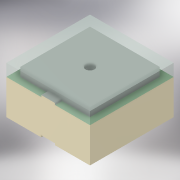
# Autodesk Inventor part: 13360-30xxVE
Saved by Autodesk Inventor 2019 (Build 230136000, 136)
## iProperties
Created: 2016-06-07
Part Number: 13360-30xxVE
Material: ABS Plastic
Document SubType Name: Modeling
Designer: sawaiz
Density: 1.06 g/cm^3
Appearance: Smooth - White
Author: sawaiz
Autodesk Inventor part; units mm, degrees
ref_plane "YZ Plane" through (0, 0, 0) normal (1, 0, 0) x (0, 1, 0)
ref_plane "XZ Plane" through (0, 0, 0) normal (0, 1, 0) x (-1, 0, 0)
ref_plane "XY Plane" through (0, 0, 0) normal (0, 0, 1) x (1, 0, 0)
sketch "Sketch1" plane through (0, 0, 0) normal (0, 1, 0) x (-1, 0, 0)
  line L0 (1.2, 1.2) -> (-1.2, 1.2)
  line L1 (-1.2, 1.2) -> (-1.2, -1.2)
  line L2 (-1.2, -1.2) -> (1.2, -1.2)
  line L3 (1.2, -1.2) -> (1.2, 1.2)
  line L4 (1.2, 1.2) -> (-1.2, -1.2) construction
  line L5 (-1.2, 1.2) -> (1.2, -1.2) construction
  point P0 (0, 0)
  dimension "d0" = 2.4
  dimension "d1" = 2.4
  constraints: 12 end point, 2 midpoint, 2 parallel, 1 horizontal, 1 perpendicular
  measures "d0" distance of L2.end L1.end
  measures "d1" distance of L1.end L0.end
extrude "Extrusion1" add sketch "Sketch1" along normal blind 1
sketch "Sketch2" plane through (0, 1, 0) normal (0, 1, 0) x (1, 0, 0)
  line L0 (1, -1) -> (-1, -1)
  line L1 (-1, -1) -> (-1, 1)
  line L2 (-1, 1) -> (1, 1)
  line L3 (1, 1) -> (1, -1)
  line L4 (1, -1) -> (-1, 1) construction
  line L5 (-1, -1) -> (1, 1) construction
  point P0 (0, 0)
  dimension "d4" = 2
  dimension "d5" = 2
  constraints: 12 end point, 2 midpoint, 2 parallel, 1 horizontal, 1 perpendicular
  measures "d4" distance of L1.end L2.end
  measures "d5" distance of L0.end L1.end
extrude "Extrusion2" add sketch "Sketch2" along normal blind 0.25 separate body
sketch "Sketch8" plane through (0, 1, 0) normal (0, 1, 0) x (1, 0, 0)
  line L0 (-1.2, -1.2) -> (1.2, -1.2) projected
  line L1 (1.2, -1.2) -> (1.2, 1.2) projected
  line L2 (1.2, 1.2) -> (-1.2, 1.2) projected
  line L3 (-1.2, 1.2) -> (-1.2, -1.2) projected
  line L4 (-1, -1) -> (1, -1) projected
  line L5 (-0.2, -1.2) -> (0.2, -1.2)
  line L6 (0.2, -1.2) -> (0.2, -1)
  line L7 (0.2, -1) -> (-0.2, -1)
  line L8 (-0.2, -1) -> (-0.2, -1.2)
  point P0 (0, 0)
  point P1 (0, -1)
  point P2 (0, -1.2)
  dimension "d49" = 0.4
  constraints: 8 end point, 3 midpoint, 2 parallel, 2 point on line, 1 horizontal, 1 perpendicular
  measures "d49" distance between parallel lines of L8 L6
extrude "Extrusion6" add sketch "Sketch8" along normal blind 0.05 contours L8 L4 L6 L0 bodies 1
sketch "Sketch3" plane through (0, 1, 0) normal (0, 1, 0) x (1, 0, 0)
  line L0 (-1.2, -1.2) -> (-0.2, -1.2) projected
  line L1 (1.2, -1.2) -> (1.2, 1.2) projected
  line L2 (1.2, 1.2) -> (-1.2, 1.2) projected
  line L3 (-1.2, 1.2) -> (-1.2, -1.2) projected
  line L4 (-1, -1) -> (1, -1) projected
  line L5 (1, -1) -> (1, 1) projected
  line L6 (1, 1) -> (-1, 1) projected
  line L7 (-1, 1) -> (-1, -1) projected
  line L8 (0.2, -1) -> (0.2, -1.2) projected
  line L9 (0.2, -1.2) -> (1.2, -1.2) projected
  line L10 (-0.2, -1.2) -> (-0.2, -1) projected
  line L11 (-0.2, -1) -> (0.2, -1) projected
  point P0 (0, 0)
extrude "Extrusion3" add sketch "Sketch3" along normal blind 0.35 separate body contours L3 L2 L1 L9 L8 L4 L5 L6 L7 L10 L0
sketch "Sketch9" plane through (0, 1.05, 0) normal (0, 1, 0) x (1, 0, 0)
  point P0 (0, 0)
sketch "Sketch10" plane through (0, 1.35, 0) normal (0, 1, 0) x (1, 0, 0)
  line L0 (-0.2, -1.2) -> (0.2, -1.2) projected
  line L1 (0.2, -1.2) -> (0.2, -1) projected
  line L2 (0.2, -1) -> (-0.2, -1) projected
  line L3 (-0.2, -1) -> (-0.2, -1.2) projected
  point P0 (0, 0)
extrude "Extrusion7" add sketch "Sketch10" against normal up to surface (0.3 mm away) bodies 3
sketch "Sketch5" plane through (0, 1.25, 0) normal (0, 1, 0) x (1, 0, 0)
  point P0 (0, 0)
  point P1 (0, 0)
  constraints: 1 coincident
hole "Hole1" at (0, 1.25, 0) direction (0, -1, 0) diameter 0.254 depth 0.1 tip angle 118 bodies 2
sketch "Sketch4" plane through (0, 1.35, 0) normal (0, 1, 0) x (1, 0, 0)
  line L0 (-1, -1) -> (-1, 1) projected
  line L1 (-1, 1) -> (1, 1) projected
  line L2 (1, 1) -> (1, -1) projected
  line L3 (1, -1) -> (-1, -1) projected
  line L4 (1.2, -1.2) -> (1.2, 1.2) projected
  line L5 (1.2, 1.2) -> (-1.2, 1.2) projected
  line L6 (-1.2, 1.2) -> (-1.2, -1.2) projected
  line L7 (-1.2, -1.2) -> (1.2, -1.2) projected
  point P0 (0, 0)
extrude "Extrusion4" add sketch "Sketch4" against normal up to surface (0.1 mm away) contours L0 L1 L2 L3 bodies 3
sketch "Sketch6" plane through (0, 0, 0) normal (0, -1, 0) x (1, 0, 0)
  line L0 (0.6, 0.6) -> (-0.6, 0.6)
  line L1 (-0.6, 0.6) -> (-0.6, -0.6)
  line L2 (-0.6, -0.6) -> (0.6, -0.6)
  line L3 (0.6, -0.6) -> (0.6, 0.6)
  line L4 (0.6, 0.6) -> (-0.6, -0.6) construction
  line L5 (-0.6, 0.6) -> (0.6, -0.6) construction
  point P0 (0, 0)
  point P1 (0, 0)
  point P2 (0, 0)
  dimension "d19" = 1.2
  dimension "d20" = 1.2
  constraints: 12 end point, 4 coincident, 2 midpoint, 2 parallel, 1 horizontal, 1 perpendicular
  measures "d19" distance of L2.end L1.end
  measures "d20" distance of L1.end L0.end
hole "Hole2" at (0.6, 0, -0.6) at (-0.6, 0, -0.6) at (0.6, 0, 0.6) at (-0.6, 0, 0.6) direction (0, 1, 0) diameter 0.8 depth 0.05 bodies 1
sketch "Sketch11" plane through (0, 0, 0) normal (0, -1, 0) x (1, 0, 0)
  circle A0 centre (0.6, -0.6) radius 0.4 projected
  circle A1 centre (-0.6, -0.6) radius 0.4 projected
  circle A2 centre (0.6, 0.6) radius 0.4 projected
  line L0 (-1.2, 1.2) -> (1.2, 1.2) projected
  line L1 (-1.2, -1.2) -> (-1.2, 1.2) projected
  line L2 (1.2, -1.2) -> (-1.2, -1.2) projected
  line L3 (1.2, 1.2) -> (1.2, -1.2) projected
  line L4 (0.2, 1.2) -> (-0.2, 1.2)
  line L5 (-0.2, 1.2) -> (-0.2, 1)
  line L6 (-0.2, 1) -> (0.2, 1)
  line L7 (0.2, 1) -> (0.2, 1.2)
  line L8 (-1.2, 1.2) -> (1.2, 1.2) projected
  point P0 (0, 0)
  point P1 (0, 1.2)
  point P2 (0, 1.2)
  dimension "d41" = 0.4
  dimension "d42" = 0.2
  constraints: 8 end point, 3 midpoint, 2 parallel, 1 horizontal, 1 perpendicular, 1 point on line
  measures "d41" distance of L5.end L6.end
  measures "d42" distance of L4.end L5.end
extrude "Extrusion8" cut sketch "Sketch11" against normal blind 0.05 contours L0 L7 L6 L5 bodies 1
sketch "Sketch12" plane through (0.6, 0.05, -0.6) normal (0, -1, 0) x (1, 0, 0)
  circle A0 centre (0, 0) radius 0.4 projected
  circle A1 centre (-1.2, 0) radius 0.4 projected
  circle A2 centre (0, 1.2) radius 0.4 projected
  circle A3 centre (-1.2, 1.2) radius 0.4 projected
  circle A4 centre (0, 0) radius 0.3
  circle A5 centre (-1.2, 0) radius 0.3
  circle A6 centre (-1.2, 1.2) radius 0.3
  circle A7 centre (0, 1.2) radius 0.3
  dimension "d46" = 0.6
  constraints: 4 centre point, 4 coincident, 3 equal radius
  measures "d46" diameter of A4
extrude "Extrusion9" add sketch "Sketch12" along normal up to surface (0.05 mm away) separate body contours A4 | A5 | A6 | A7
body "Solid1"
body "Solid2"
body "Solid3"
body "Solid5"
